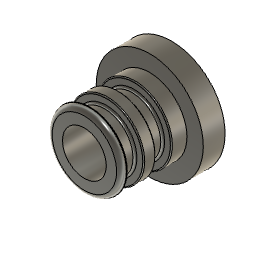
D100 v3 (Autodesk Fusion 360 design; units mm, degrees)
Autodesk Fusion 360 part; units mm, degrees
sketch "Sketch1" plane through (0, 0, 0) normal (0, 0, 1) x (1, 0, 0)
  line L0 (99.1556, 117.5621) -> (99.1556, 25) construction
  line L1 (106.8056, 112) -> (106.8056, 109)
  line L2 (106.8056, 112) -> (110.1556, 112)
  line L3 (105.0056, 108.4) -> (105.0056, 106)
  line L4 (105.4056, 108.8) -> (106.6056, 108.8)
  line L5 (105.4056, 105.6) -> (106.6056, 105.6)
  line L6 (106.8056, 105.4) -> (106.8056, 103.3)
  line L7 (106.6056, 103.1) -> (105.4056, 103.1)
  line L8 (105.0056, 102.7) -> (105.0056, 100.3)
  line L9 (105.4056, 99.9) -> (106.6056, 99.9)
  line L10 (106.8056, 99.7) -> (106.8056, 99.5492)
  line L11 (105.2556, 116.5) -> (105.2556, 116)
  line L12 (105.2556, 116) -> (105.2556, 111)
  line L13 (105.2556, 111) -> (103.657, 111)
  line L14 (103.657, 111) -> (103.6567, 99.5621)
  arc A0 (105.4056, 108.8) -> (105.0056, 108.4) centre (105.4056, 108.4) ccw
  arc A1 (105.0056, 106) -> (105.4056, 105.6) centre (105.4056, 106) ccw
  arc A2 (105.4056, 103.1) -> (105.0056, 102.7) centre (105.4056, 102.7) ccw
  arc A3 (105.0056, 100.3) -> (105.4056, 99.9) centre (105.4056, 100.3) ccw
  line L15 (110.1556, 112) -> (110.1556, 112.4941)
  line L16 (110.1556, 112.4941) -> (110.1556, 116.4941)
  line L17 (110.1556, 116.4941) -> (105.2556, 116.5)
  line L18 (103.6567, 98.5492) -> (103.6567, 99.5621)
  arc A4 (106.8056, 99.7) -> (106.6056, 99.9) centre (106.6056, 99.7) ccw
  arc A5 (106.8056, 105.4) -> (106.6056, 105.6) centre (106.6056, 105.4) ccw
  arc A6 (106.6056, 103.1) -> (106.8056, 103.3) centre (106.6056, 103.3) ccw
  arc A7 (106.6056, 108.8) -> (106.8056, 109) centre (106.6056, 109) ccw
  arc A8 (105.7927, 98.5492) -> (106.8056, 99.5621) centre (105.7928, 99.5621) ccw
  line L19 (103.6567, 98.5492) -> (105.7927, 98.5492)
  point P0 (106.8056, 108.8)
  point P1 (105.0056, 108.8)
  point P2 (105.0056, 105.6)
  point P3 (105.0056, 103.1)
  point P4 (105.0056, 99.9)
  dimension "d5" = 3.2
  dimension "d7" = 3.2
  dimension "d9" = 3.2
  dimension "d14" = 5
  dimension "d16" = 0.4
  dimension "d17" = 0.4
  dimension "d18" = 0.4
  dimension "d19" = 0.4
  dimension "d20" = 4
  dimension "d22" = 0.2
  dimension "d23" = 0.2
  dimension "d24" = 0.2
  dimension "d25" = 0.2
  constraint vertical L0
  constraint perpendicular L1 L4
  constraint perpendicular L3 L5
  constraint perpendicular L5 L6
  constraint perpendicular L3 L7
  constraint perpendicular L7 L8
  constraint perpendicular L6 L9
  constraint perpendicular L9 L10
  constraint perpendicular L0 L13
  constraint coincident P1 L4
  constraint coincident P1 L3
  constraint tangent L4 A0
  constraint tangent L3 A0
  constraint coincident P2 L3
  constraint coincident P2 L5
  constraint tangent L3 A1
  constraint tangent L5 A1
  constraint coincident P3 L7
  constraint coincident P3 L8
  constraint tangent L7 A2
  constraint tangent L8 A2
  constraint coincident P4 L8
  constraint coincident P4 L9
  constraint tangent L8 A3
  constraint tangent L9 A3
  constraint perpendicular L2 L15
  constraint parallel L15 L16
  constraint tangent L9 A4
  constraint tangent L10 A4
  constraint tangent L5 A5
  constraint tangent L6 A5
  constraint tangent L6 A6
  constraint tangent L7 A6
  constraint coincident P0 L1
  constraint coincident P0 L4
  constraint tangent L1 A7
  constraint tangent L4 A7
  constraint tangent L10 A8
  constraint coincident L10 A8.end
  constraint perpendicular L18 L19
  measures "d5" distance of L1.start P0
  measures "d7" distance of P1 P2
  measures "d9" distance of P3 P4
  measures "d14" distance of L11.end L12.end
  measures "d16" radius of A0
  measures "d17" radius of A1
  measures "d18" radius of A2
  measures "d19" radius of A3
  measures "d20" distance of L15.end L16.end
  measures "d22" radius of A4
  measures "d23" radius of A5
  measures "d24" radius of A6
  measures "d25" radius of A7
revolve "Revolve1" add sketch "Sketch1" angle 360 about axis through (99.1556, 117.5621, 0) along (0, -1, 0)
